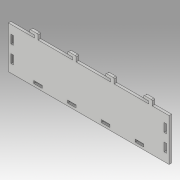
# Autodesk Inventor part: long_side1
Saved by Autodesk Inventor 2019.3 (Build 233278000, 278)
## iProperties
Created: 2019-06-26
Part Number: long_side1
Material: Generic
Document SubType Name: Modeling
Designer: Dave
Density: 1 g/cm^3
Appearance: Default
Author: Dave
Autodesk Inventor part; units mm, degrees
ref_plane "YZ Plane" through (0, 0, 0) normal (1, 0, 0) x (0, 1, 0)
ref_plane "XZ Plane" through (0, 0, 0) normal (0, 1, 0) x (-1, 0, 0)
ref_plane "XY Plane" through (0, 0, 0) normal (0, 0, 1) x (1, 0, 0)
sketch "Sketch1" plane through (0, 0, 0) normal (0, 0, 1) x (1, 0, 0)
  line L0 (0, 0) -> (190, 0)
  line L1 (190, 0) -> (190, 50)
  line L2 (0, 50) -> (0, 0)
  line L3 (31, 50) -> (31, 53)
  line L4 (31, 53) -> (26, 53)
  line L5 (25, 54) -> (25, 55)
  line L6 (26, 56) -> (34, 56)
  line L7 (35, 55) -> (35, 50)
  line L8 (76, 50) -> (76, 53)
  line L9 (76, 53) -> (71, 53)
  line L10 (70, 54) -> (70, 55)
  line L11 (71, 56) -> (79, 56)
  line L12 (80, 55) -> (80, 50)
  line L13 (121, 50) -> (121, 53)
  line L14 (121, 53) -> (116, 53)
  line L15 (115, 54) -> (115, 55)
  line L16 (116, 56) -> (124, 56)
  line L17 (125, 55) -> (125, 50)
  line L18 (166, 50) -> (166, 53)
  line L19 (166, 53) -> (161, 53)
  line L20 (160, 54) -> (160, 55)
  line L21 (161, 56) -> (169, 56)
  line L22 (170, 55) -> (170, 50)
  arc A0 (26, 56) -> (25, 55) centre (26, 55) ccw
  arc A1 (25, 54) -> (26, 53) centre (26, 54) ccw
  arc A2 (35, 55) -> (34, 56) centre (34, 55) ccw
  arc A3 (70, 54) -> (71, 53) centre (71, 54) ccw
  arc A4 (71, 56) -> (70, 55) centre (71, 55) ccw
  arc A5 (80, 55) -> (79, 56) centre (79, 55) ccw
  arc A6 (116, 56) -> (115, 55) centre (116, 55) ccw
  arc A7 (115, 54) -> (116, 53) centre (116, 54) ccw
  arc A8 (125, 55) -> (124, 56) centre (124, 55) ccw
  arc A9 (161, 56) -> (160, 55) centre (161, 55) ccw
  arc A10 (160, 54) -> (161, 53) centre (161, 54) ccw
  arc A11 (170, 55) -> (169, 56) centre (169, 55) ccw
  line L23 (31, 50) -> (0, 50)
  line L24 (76, 50) -> (35, 50)
  line L25 (121, 50) -> (80, 50)
  line L26 (190, 50) -> (170, 50)
  line L27 (166, 50) -> (125, 50)
  line L28 (3, 40) -> (6, 40)
  line L29 (6, 40) -> (6, 30)
  line L30 (6, 30) -> (3, 30)
  line L31 (3, 30) -> (3, 40)
  line L32 (3, 20) -> (6, 20)
  line L33 (6, 20) -> (6, 10)
  line L34 (6, 10) -> (3, 10)
  line L35 (3, 10) -> (3, 20)
  line L36 (184, 40) -> (187, 40)
  line L37 (187, 40) -> (187, 30)
  line L38 (187, 30) -> (184, 30)
  line L39 (184, 30) -> (184, 40)
  line L40 (184, 20) -> (187, 20)
  line L41 (187, 20) -> (187, 10)
  line L42 (187, 10) -> (184, 10)
  line L43 (184, 10) -> (184, 20)
  line L44 (30, 6) -> (40, 6)
  line L45 (40, 6) -> (40, 3)
  line L46 (40, 3) -> (30, 3)
  line L47 (30, 3) -> (30, 6)
  line L48 (70, 6) -> (80, 6)
  line L49 (80, 6) -> (80, 3)
  line L50 (80, 3) -> (70, 3)
  line L51 (70, 3) -> (70, 6)
  line L52 (110, 6) -> (120, 6)
  line L53 (120, 6) -> (120, 3)
  line L54 (120, 3) -> (110, 3)
  line L55 (110, 3) -> (110, 6)
  line L56 (150, 6) -> (160, 6)
  line L57 (160, 6) -> (160, 3)
  line L58 (160, 3) -> (150, 3)
  line L59 (150, 3) -> (150, 6)
  point P0 (25, 53)
  point P1 (25, 56)
  point P2 (35, 56)
  point P3 (70, 53)
  point P4 (70, 56)
  point P5 (80, 56)
  point P6 (115, 53)
  point P7 (115, 56)
  point P8 (125, 56)
  point P9 (160, 53)
  point P10 (160, 56)
  point P11 (170, 56)
  point P12 (190, 25)
  point P13 (0, 25)
  dimension "d6" = 190
  dimension "d7" = 50
  dimension "d19" = 20
  dimension "d23" = 10
  dimension "d24" = 3
  dimension "d25" = 3
  dimension "d26" = 4
  dimension "d27" = 1
  dimension "d28" = 45
  dimension "d29" = 45
  dimension "d30" = 45
  dimension "d31" = 31
  dimension "d34" = 3
  dimension "d35" = 10
  dimension "d36" = 10
  dimension "d37" = 3
  dimension "d51" = 10
  dimension "d52" = 30
  dimension "d53" = 30
  dimension "d54" = 30
  dimension "d55" = 30
  dimension "d56" = 3
  dimension "d57" = 3
  dimension "d60" = 10
  dimension "d61" = 3
  constraints: 120 end point, 50 point on line, 45 perpendicular, 24 parallel, 24 point on circle, 24 tangent, 12 centre point, 11 equal length, 11 equal radius, 9 horizontal, 3 collinear, 2 midpoint
  measures "d6" distance of L1.end L2.start
  measures "d7" distance of L0.end L1.end
  measures "d19" distance between parallel lines of L22 L1
  measures "d23" distance of point (25, 56) point (35, 56)
  measures "d24" distance of L3.start L3.end
  measures "d25" distance of point (25, 53) point (25, 56)
  measures "d26" distance between parallel lines of L7 L3
  measures "d27" radius of A0
  measures "d28" distance between parallel lines of L17 L22
  measures "d29" distance between parallel lines of L12 L17
  measures "d30" distance between parallel lines of L7 L12
  measures "d31" distance of L3.start L2.start
  measures "d34" distance between parallel lines of L2 L31
  measures "d35" distance between parallel lines of L0 L34
  measures "d36" distance between parallel lines of L23 L28
  measures "d37" distance between parallel lines of L1 L37
  measures "d51" distance of L45.end L46.end
  measures "d52" distance between parallel lines of L57 L1
  measures "d53" distance between parallel lines of L2 L47
  measures "d54" distance between parallel lines of L59 L53
  measures "d55" distance between parallel lines of L51 L45
  measures "d56" distance between parallel lines of L0 L50
  measures "d57" distance of L44.end L45.end
  measures "d60" distance of L28.end L29.end
  measures "d61" distance of L29.end L30.end
extrude "Extrusion3" add sketch "Sketch1" along normal blind 3
body "Solid3"
